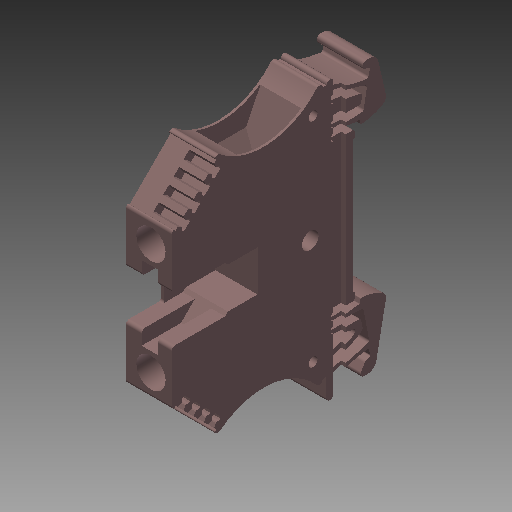
# Autodesk Inventor part: WDU 10 1020300000
Saved by Autodesk Inventor 2019.3 (Build 233278000, 278)
## iProperties
Category: PARTsolutions
Company: WEIDMUELLER
Created: 2018-11-07
Part Number: WDU 10 1020300000
Material: Generic
Catalog Web Link: www.cadenas.de
Description: WDU 10-Feed Through Terminal
Vendor: WEIDMUELLER
Document SubType Name: Modeling
Designer: psadmin
Manufacturer: WEIDMUELLER
Mass: 15.1532 g
Surface Area: 85.6547 cm^2
Volume: 15.1532 cm^3
Density: 1 g/cm^3
Appearance: PSOLRGB-175-140-135
PSOL_IDENT_0: {$CADENAS_DATA\23d-libs\weidmueller\reihenklemmen\w_series\durchgangs_rk\wdu10.prj},174 {VTYP=3D},{N
PSOL_IDENT_1: B=WDU 10 1020300000},{LINA=WDU 10 1020300000},{NN=WDU 10},{DATE=31.03.2017 09:23:17},{GEOMDATE=27.10
PSOL_IDENT_2: .2015 08:25:59},{VERSION=},{LINEID=10},{WBVAR=},{WBNUMERIC=}  {NB=WDU 10 1020300000},{LINA=WDU 10 10
PSOL_IDENT_3: 20300000},{KT=DUMMY},{BEST=1020300000},{BZ=WDU 10},{M=Wemid},{F=beige},{FCODE=0.69,0.55,0.53,0.00}
NN: WDU 10
NT: Feed Through Terminal
NB: WDU 10 1020300000
NBSYN: $BZ. $BEST.
LINA: WDU 10 1020300000
BEST: 1020300000
BZ: WDU 10
M: Wemid
F: beige
SUPPLIER: WEIDMUELLER
ARTICLENO: WDU 10 1020300000
BOMINFO: WDU 10 1020300000
CREATOR: CADENAS GmbH
Title: WDU 10 1020300000
Author: Cadenas PARTsolutions
Comments: Feed Through Terminal
Autodesk Inventor part; units mm, degrees
ref_plane "YZ Plane" through (0, 0, 0) normal (1, 0, 0) x (0, 1, 0)
ref_plane "XZ Plane" through (0, 0, 0) normal (0, 1, 0) x (-1, 0, 0)
ref_plane "XY Plane" through (0, 0, 0) normal (0, 0, 1) x (1, 0, 0)
sketch "Sketch_1" plane through (0, 0, 0) normal (1, 0, 0) x (0, 1, 0)
  line L0 (48.05, 46.25) -> (37.75, 46.25)
  arc A0 (37.75, 46.25) -> (37, 45.5) centre (37.75, 45.5) ccw
  line L1 (37, 45.5) -> (37, 39.25)
  arc A1 (36.5, 38.75) -> (37, 39.25) centre (36.5, 39.25) ccw
  line L2 (36.5, 38.75) -> (27.5, 38.75)
  arc A2 (27, 39.25) -> (27.5, 38.75) centre (27.5, 39.25) ccw
  line L3 (27, 39.25) -> (27, 45.5)
  arc A3 (27, 45.5) -> (26.25, 46.25) centre (26.25, 45.5) ccw
  line L4 (26.25, 46.25) -> (15.95, 46.25)
  arc A4 (15.95, 46.25) -> (15.4144, 46.0251) centre (15.95, 45.5) ccw
  arc A5 (15.4144, 46.0251) -> (15.4159, 45.673) centre (15.5927, 45.8497) ccw
  line L5 (15.4159, 45.673) -> (15.6294, 45.4594)
  line L6 (15.6294, 45.4594) -> (6.7906, 36.6206)
  line L7 (6.7906, 36.6206) -> (6.577, 36.8341)
  arc A6 (6.577, 36.8341) -> (6.2256, 36.8362) centre (6.4003, 36.6573) ccw
  arc A7 (6.2256, 36.8362) -> (6.1668, 35.8284) centre (6.75, 36.3) ccw
  arc A8 (4.2611, 14.9688) -> (6.1668, 35.8284) centre (-5.5492, 26.3819) ccw
  arc A9 (4.2611, 14.9688) -> (4.75, 13.65) centre (4.75, 14.4) ccw
  line L8 (4.75, 13.65) -> (4.75, 12.9)
  line L9 (4.75, 12.9) -> (0.75, 12.9)
  arc A10 (0.75, 12.9) -> (0.4862, 11.4479) centre (0.75, 12.15) ccw
  line L10 (0.4862, 11.4479) -> (1.9437, 10.9003)
  line L11 (1.9437, 10.9003) -> (3.401, 10.9003)
  arc A11 (3.8733, 10.5645) -> (3.401, 10.9003) centre (3.401, 10.4003) ccw
  arc A12 (5.4944, 4.2319) -> (3.8733, 10.5645) centre (-33.9366, -2.4884) ccw
  arc A13 (5.333, 3.774) -> (5.4944, 4.2319) centre (5.0014, 4.1482) ccw
  arc A14 (5.2197, 3.7112) -> (5.333, 3.774) centre (5.1344, 3.9988) ccw
  line L12 (5.2197, 3.7112) -> (4.167, 3.399)
  arc A15 (3.9289, 3.5062) -> (4.167, 3.399) centre (4.1102, 3.5908) ccw
  line L13 (3.9289, 3.5062) -> (3.559, 4.299)
  arc A16 (3.559, 4.299) -> (3.255, 4.632) centre (2.8787, 3.9832) ccw
  line L14 (3.255, 4.632) -> (1.925, 5.4)
  arc A17 (1.925, 5.4) -> (0.8, 4.7505) centre (1.55, 4.7505) ccw
  line L15 (0.8, 4.7505) -> (0.8, 4.05)
  arc A18 (0.8, 4.05) -> (2.4156, 2.0873) centre (2.8, 4.05) ccw
  line L16 (2.4156, 2.0873) -> (12.9502, 0.0242)
  arc A19 (12.9502, 0.0242) -> (14.303, 0.6119) centre (13.2, 1.3) ccw
  arc A20 (14.303, 0.6119) -> (15.7996, 5.2872) centre (5.8187, 5.905) ccw
  arc A21 (15.7996, 5.2872) -> (15.6552, 5.4922) centre (15.6, 5.2999) ccw
  line L17 (15.6552, 5.4922) -> (14.9048, 5.7077)
  arc A22 (14.76, 5.9) -> (14.9048, 5.7077) centre (14.96, 5.9) ccw
  line L18 (14.76, 5.9) -> (14.76, 6.75)
  arc A23 (14.5026, 11.4514) -> (14.76, 6.75) centre (29.4233, 9.9104) ccw
  arc A24 (15, 11.9) -> (14.5026, 11.4514) centre (15, 11.4) ccw
  line L19 (15, 11.9) -> (15.5, 11.9)
  arc A25 (16, 11.4) -> (15.5, 11.9) centre (15.5, 11.4) ccw
  line L20 (16, 11.4) -> (16, 7.25)
  arc A26 (16, 7.25) -> (16.5, 6.75) centre (16.5, 7.25) ccw
  line L21 (16.5, 6.75) -> (17.5, 6.75)
  line L22 (17.5, 6.75) -> (17.8, 7.05)
  line L23 (17.8, 7.05) -> (46.2, 7.05)
  line L24 (46.2, 7.05) -> (46.5, 6.75)
  line L25 (46.5, 6.75) -> (47.5, 6.75)
  arc A27 (47.5, 6.75) -> (48, 7.25) centre (47.5, 7.25) ccw
  line L26 (48, 7.25) -> (48, 11.4)
  arc A28 (48.5, 11.9) -> (48, 11.4) centre (48.5, 11.4) ccw
  line L27 (48.5, 11.9) -> (49, 11.9)
  arc A29 (49.4974, 11.4509) -> (49, 11.9) centre (49, 11.4) ccw
  arc A30 (49.24, 6.7494) -> (49.4974, 11.4509) centre (34.5768, 9.91) ccw
  line L28 (49.24, 6.7494) -> (49.24, 5.9)
  arc A31 (49.0952, 5.7078) -> (49.24, 5.9) centre (49.04, 5.9) ccw
  line L29 (49.0952, 5.7078) -> (48.3444, 5.4921)
  arc A32 (48.3444, 5.4921) -> (48.2004, 5.2878) centre (48.3995, 5.3003) ccw
  arc A33 (48.2004, 5.2878) -> (49.697, 0.6119) centre (58.1813, 5.905) ccw
  arc A34 (49.697, 0.6119) -> (51.0937, 0.0336) centre (50.8, 1.3) ccw
  line L30 (51.0937, 0.0336) -> (58.147, 1.6508)
  arc A35 (58.147, 1.6508) -> (59.7, 3.6004) centre (57.7, 3.6002) ccw
  line L31 (59.7, 3.6004) -> (59.7, 4.25)
  arc A36 (59.7, 4.25) -> (58.95, 5) centre (58.95, 4.25) ccw
  line L32 (58.95, 5) -> (58.6838, 5)
  arc A37 (58.6838, 5) -> (58.2009, 4.6297) centre (58.6838, 4.5) ccw
  line L33 (58.2009, 4.6297) -> (57.9338, 3.6353)
  arc A38 (57.697, 3.492) -> (57.9338, 3.6353) centre (57.7407, 3.6872) ccw
  line L34 (57.697, 3.492) -> (56.4904, 3.762)
  arc A39 (56.1072, 4.3347) -> (56.4904, 3.762) centre (56.6, 4.2499) ccw
  arc A40 (57.8794, 11.0689) -> (56.1072, 4.3347) centre (95.5295, -2.4393) ccw
  arc A41 (58.35, 11.4) -> (57.8794, 11.0689) centre (58.35, 10.9) ccw
  line L35 (58.35, 11.4) -> (59.25, 11.4)
  arc A42 (59.25, 11.4) -> (59.25, 12.9) centre (59.25, 12.15) ccw
  line L36 (59.25, 12.9) -> (59.25, 13.65)
  arc A43 (59.25, 13.65) -> (59.7395, 14.9682) centre (59.25, 14.4) ccw
  arc A44 (57.8338, 35.8292) -> (59.7395, 14.9682) centre (69.5492, 26.3819) ccw
  arc A45 (57.8338, 35.8292) -> (57.7746, 36.836) centre (57.25, 36.3) ccw
  arc A46 (57.7746, 36.836) -> (57.423, 36.8341) centre (57.5997, 36.6573) ccw
  line L37 (57.423, 36.8341) -> (57.2094, 36.6206)
  line L38 (57.2094, 36.6206) -> (48.3706, 45.4594)
  line L39 (48.3706, 45.4594) -> (48.5841, 45.673)
  arc A47 (48.5841, 45.673) -> (48.5856, 46.0251) centre (48.4073, 45.8497) ccw
  arc A48 (48.5856, 46.0251) -> (48.05, 46.25) centre (48.05, 45.5) ccw
  arc A49 (8.5, 11.4) -> (8.0182, 10.7663) centre (8.5, 10.9) ccw
  arc A50 (8.0182, 10.7663) -> (9.6067, 7.0644) centre (22.4721, 14.7768) ccw
  arc A51 (9.6067, 7.0644) -> (10.8714, 7.0301) centre (10.25, 7.45) ccw
  arc A52 (11, 7.9696) -> (10.8714, 7.0301) centre (11.3, 7.45) ccw
  line L40 (11, 7.9696) -> (11, 10.9)
  arc A53 (11, 10.9) -> (10.5, 11.4) centre (10.5, 10.9) ccw
  line L41 (10.5, 11.4) -> (8.5, 11.4)
  arc A54 (55.55, 11.9) -> (55.0535, 11.4588) centre (55.55, 11.4) ccw
  arc A55 (53.9858, 5.5317) -> (55.0535, 11.4588) centre (5.4009, 17.3431) ccw
  arc A56 (53.4019, 5.1597) -> (53.9858, 5.5317) centre (53.5, 5.65) ccw
  line L42 (53.4019, 5.1597) -> (52.4019, 5.3597)
  arc A57 (52, 5.85) -> (52.4019, 5.3597) centre (52.5, 5.85) ccw
  line L43 (52, 5.85) -> (52, 11.4)
  arc A58 (52, 11.4) -> (51.5, 11.9) centre (51.5, 11.4) ccw
  line L44 (51.5, 11.9) -> (51.0523, 11.9)
  arc A59 (51.0523, 11.9) -> (50.5585, 11.4781) centre (51.0523, 11.4) ccw
  arc A60 (50.5585, 11.4781) -> (50.4084, 5.257) centre (73.7984, 7.8051) ccw
  arc A61 (50.4084, 5.257) -> (50.8126, 4.8199) centre (50.9055, 5.3112) ccw
  line L45 (50.8126, 4.8199) -> (54.4786, 4.1269)
  arc A62 (54.4786, 4.1269) -> (55.0409, 4.4461) centre (54.5714, 4.6182) ccw
  arc A63 (55.0409, 4.4461) -> (56.8124, 11.3239) centre (21.3911, 16.7805) ccw
  arc A64 (56.8124, 11.3239) -> (56.3182, 11.9) centre (56.3182, 11.4) ccw
  line L46 (56.3182, 11.9) -> (55.55, 11.9)
  arc A65 (12.5, 11.9) -> (12, 11.4) centre (12.5, 11.4) ccw
  line L47 (12, 11.4) -> (12, 5.85)
  arc A66 (11.5921, 5.3586) -> (12, 5.85) centre (11.5, 5.85) ccw
  line L48 (11.5921, 5.3586) -> (9.9921, 5.0586)
  arc A67 (9.4818, 5.2759) -> (9.9921, 5.0586) centre (9.9, 5.55) ccw
  arc A68 (7.0291, 10.543) -> (9.4818, 5.2759) centre (26.1938, 16.2627) ccw
  arc A69 (7.0291, 10.543) -> (6.55, 10.9) centre (6.55, 10.4) ccw
  line L49 (6.55, 10.9) -> (5.3694, 10.9)
  arc A70 (5.3694, 10.9) -> (4.8818, 10.2893) centre (5.3694, 10.4) ccw
  arc A71 (4.8818, 10.2893) -> (6.5858, 4.0374) centre (78.6169, 27.0276) ccw
  arc A72 (6.5858, 4.0374) -> (7.1536, 3.6979) centre (7.0621, 4.1895) ccw
  line L50 (7.1536, 3.6979) -> (13.1856, 4.8201)
  arc A73 (13.1856, 4.8201) -> (13.5912, 5.2575) centre (13.0941, 5.3117) ccw
  arc A74 (13.5912, 5.2575) -> (13.4421, 11.478) centre (-9.7985, 7.8091) ccw
  arc A75 (13.4421, 11.478) -> (12.9482, 11.9) centre (12.9482, 11.4) ccw
  line L51 (12.9482, 11.9) -> (12.5, 11.9)
  constraints: 152 point on circle, 104 end point, 76 centre point
extrude "Extrusion1" add sketch "Sketch_1" along normal blind 9.9
sketch "Skizze_2" plane through (5.4, 0, 0) normal (1, 0, 0) x (0, 0, -1)
  line L0 (-46.75, 20) -> (-38.75, 20)
  line L1 (-38.75, 20) -> (-38.75, 16.84)
  line L2 (-38.75, 16.84) -> (-46.75, 16.84)
  line L3 (-46.75, 16.84) -> (-46.75, 20)
  line L4 (-46.75, 20) -> (-38.75, 20)
  constraints: 10 end point
revolve "Revolution1" cut sketch "Skizze_2" angle 360 about axis through (5.4, 20, 46.75) along (0, 0, 1)
sketch "Skizze_3" plane through (5.4, 0, 0) normal (1, 0, 0) x (0, 0, -1)
  line L0 (-46.75, 44) -> (-38.75, 44)
  line L1 (-38.75, 44) -> (-38.75, 40.84)
  line L2 (-38.75, 40.84) -> (-46.75, 40.84)
  line L3 (-46.75, 40.84) -> (-46.75, 44)
  line L4 (-46.75, 44) -> (-38.75, 44)
  constraints: 10 end point
revolve "Revolution2" cut sketch "Skizze_3" angle 360 about axis through (5.4, 44, 46.75) along (0, 0, 1)
sketch "Skizze_4" plane through (0.5, 0, 0) normal (1, 0, 0) x (0, 0, -1)
  line L0 (-31.85, 55.5) -> (-26.28, 47.5)
  line L1 (-26.28, 47.5) -> (-22.38, 47.5)
  line L2 (-22.38, 47.5) -> (-17.65, 57.2)
  line L3 (-17.65, 57.2) -> (-31.85, 55.5)
  constraints: 8 end point
extrude "Extrusion2" cut sketch "Skizze_4" along normal blind 8.9
sketch "Skizze_5" plane through (0.5, 0, 0) normal (1, 0, 0) x (0, 0, -1)
  line L0 (-31.85, 8.5) -> (-17.65, 6.8)
  line L1 (-17.65, 6.8) -> (-22.38, 16.5)
  line L2 (-22.38, 16.5) -> (-26.28, 16.5)
  line L3 (-26.28, 16.5) -> (-31.85, 8.5)
  constraints: 8 end point
extrude "Extrusion3" cut sketch "Skizze_5" along normal blind 8.9
sketch "Sketch_5" plane through (0, 0, 23.45) normal (0, 0, 1) x (1, 0, 0)
  line L0 (0.3069, 14.1657) -> (0.5, 13.285)
  line L1 (0.5, 13.285) -> (6.4333, 19.2183)
  line L2 (6.4333, 19.2183) -> (9.4, 13.285)
  line L3 (9.4, 13.285) -> (9.6402, 14.1657)
  line L4 (9.6402, 14.1657) -> (9.6402, 49.3357)
  line L5 (9.6402, 49.3357) -> (9.4, 50.715)
  line L6 (9.4, 50.715) -> (6.4333, 44.7817)
  line L7 (6.4333, 44.7817) -> (0.5, 50.715)
  line L8 (0.5, 50.715) -> (0.3069, 50.0567)
  line L9 (0.3069, 50.0567) -> (0.3069, 14.1657)
  constraints: 20 end point
extrude "Extrusion4" add sketch "Sketch_5" along normal mid plane 10
sketch "Sketch_4" plane through (5.15, 0, 0) normal (1, 0, 0) x (0, 0, -1)
  line L0 (-47.25, 40) -> (-47.25, 24)
  line L1 (-47.25, 24) -> (-37.75, 24)
  line L2 (-37.75, 24) -> (-34.15, 27.6)
  line L3 (-34.15, 27.6) -> (-27.75, 27.6)
  line L4 (-27.75, 27.6) -> (-27.75, 36.4)
  line L5 (-27.75, 36.4) -> (-34.15, 36.4)
  line L6 (-34.15, 36.4) -> (-37.75, 40)
  line L7 (-37.75, 40) -> (-47.25, 40)
  constraints: 16 end point
extrude "Extrusion5" cut sketch "Sketch_4" along normal mid plane 3.55
sketch "Sketch_2" plane through (9.9, 0, 0) normal (1, 0, 0) x (0, 0, -1)
  line L0 (-47.25, 37) -> (-47.25, 27)
  line L1 (-47.25, 27) -> (-34.75, 27)
  line L2 (-34.75, 27) -> (-34.15, 27.6)
  line L3 (-34.15, 27.6) -> (-27.75, 27.6)
  line L4 (-27.75, 27.6) -> (-27.75, 36.4)
  line L5 (-27.75, 36.4) -> (-34.15, 36.4)
  line L6 (-34.15, 36.4) -> (-34.75, 37)
  line L7 (-34.75, 37) -> (-47.25, 37)
  constraints: 16 end point
extrude "Extrusion6" cut sketch "Sketch_2" against normal blind 9.1
sketch "Sketch_3" plane through (4.55, 0, 0) normal (1, 0, 0) x (0, 0, -1)
  line L0 (-50.2151, 49.9527) -> (-48.7516, 12.801)
  line L1 (-48.7516, 12.801) -> (-38.528, 4.5188)
  line L2 (-38.528, 4.5188) -> (-36.7355, 8.0369)
  line L3 (-36.7355, 8.0369) -> (-36.5941, 8.1783)
  line L4 (-36.5941, 8.1783) -> (-36.0107, 8.1783)
  line L5 (-36.0107, 8.1783) -> (-35.7721, 8.4169)
  line L6 (-35.7721, 8.4169) -> (-35.7721, 8.8412)
  line L7 (-35.7721, 8.8412) -> (-36.8327, 9.9019)
  line L8 (-36.8327, 9.9019) -> (-37.257, 9.9019)
  line L9 (-37.257, 9.9019) -> (-37.4956, 9.6632)
  line L10 (-37.4956, 9.6632) -> (-37.4956, 9.0798)
  line L11 (-37.4956, 9.0798) -> (-37.637, 8.9384)
  line L12 (-37.637, 8.9384) -> (-39.0655, 8.2106)
  line L13 (-39.0655, 8.2106) -> (-39.6679, 8.7757)
  line L14 (-39.6679, 8.7757) -> (-38.9275, 10.2289)
  line L15 (-38.9275, 10.2289) -> (-38.7861, 10.3703)
  line L16 (-38.7861, 10.3703) -> (-38.2027, 10.3703)
  line L17 (-38.2027, 10.3703) -> (-37.9641, 10.609)
  line L18 (-37.9641, 10.609) -> (-37.9641, 11.0332)
  line L19 (-37.9641, 11.0332) -> (-39.0247, 12.0939)
  line L20 (-39.0247, 12.0939) -> (-39.449, 12.0939)
  line L21 (-39.449, 12.0939) -> (-39.6877, 11.8552)
  line L22 (-39.6877, 11.8552) -> (-39.6877, 11.2719)
  line L23 (-39.6877, 11.2719) -> (-39.8291, 11.1305)
  line L24 (-39.8291, 11.1305) -> (-41.1372, 10.4639)
  line L25 (-41.1372, 10.4639) -> (-41.7545, 11.1748)
  line L26 (-41.7545, 11.1748) -> (-41.1195, 12.4209)
  line L27 (-41.1195, 12.4209) -> (-40.9781, 12.5623)
  line L28 (-40.9781, 12.5623) -> (-40.3948, 12.5623)
  line L29 (-40.3948, 12.5623) -> (-40.1561, 12.801)
  line L30 (-40.1561, 12.801) -> (-40.1561, 13.2253)
  line L31 (-40.1561, 13.2253) -> (-41.2168, 14.2859)
  line L32 (-41.2168, 14.2859) -> (-41.641, 14.2859)
  line L33 (-41.641, 14.2859) -> (-41.8797, 14.0473)
  line L34 (-41.8797, 14.0473) -> (-41.8797, 13.4639)
  line L35 (-41.8797, 13.4639) -> (-42.0211, 13.3225)
  line L36 (-42.0211, 13.3225) -> (-43.3692, 12.6356)
  line L37 (-43.3692, 12.6356) -> (-43.9752, 13.3106)
  line L38 (-43.9752, 13.3106) -> (-43.3116, 14.613)
  line L39 (-43.3116, 14.613) -> (-43.1702, 14.7544)
  line L40 (-43.1702, 14.7544) -> (-42.5868, 14.7544)
  line L41 (-42.5868, 14.7544) -> (-42.3481, 14.993)
  line L42 (-42.3481, 14.993) -> (-42.3481, 15.4173)
  line L43 (-42.3481, 15.4173) -> (-43.4088, 16.4779)
  line L44 (-43.4088, 16.4779) -> (-43.8331, 16.4779)
  line L45 (-43.8331, 16.4779) -> (-44.0717, 16.2393)
  line L46 (-44.0717, 16.2393) -> (-44.0717, 15.6559)
  line L47 (-44.0717, 15.6559) -> (-44.2131, 15.5145)
  line L48 (-44.2131, 15.5145) -> (-46.5212, 14.3385)
  line L49 (-46.5212, 14.3385) -> (-46.7415, 49.7737)
  line L50 (-46.7415, 49.7737) -> (-44.2131, 48.4855)
  line L51 (-44.2131, 48.4855) -> (-44.0717, 48.3441)
  line L52 (-44.0717, 48.3441) -> (-44.0717, 47.7607)
  line L53 (-44.0717, 47.7607) -> (-43.8331, 47.5221)
  line L54 (-43.8331, 47.5221) -> (-43.4088, 47.5221)
  line L55 (-43.4088, 47.5221) -> (-42.3481, 48.5827)
  line L56 (-42.3481, 48.5827) -> (-42.3481, 49.007)
  line L57 (-42.3481, 49.007) -> (-42.5868, 49.2456)
  line L58 (-42.5868, 49.2456) -> (-43.1702, 49.2456)
  line L59 (-43.1702, 49.2456) -> (-43.3116, 49.387)
  line L60 (-43.3116, 49.387) -> (-44.0128, 50.7632)
  line L61 (-44.0128, 50.7632) -> (-43.3726, 51.3661)
  line L62 (-43.3726, 51.3661) -> (-42.0211, 50.6775)
  line L63 (-42.0211, 50.6775) -> (-41.8797, 50.5361)
  line L64 (-41.8797, 50.5361) -> (-41.8797, 49.9527)
  line L65 (-41.8797, 49.9527) -> (-41.641, 49.7141)
  line L66 (-41.641, 49.7141) -> (-41.2168, 49.7141)
  line L67 (-41.2168, 49.7141) -> (-40.1561, 50.7747)
  line L68 (-40.1561, 50.7747) -> (-40.1561, 51.199)
  line L69 (-40.1561, 51.199) -> (-40.3948, 51.4377)
  line L70 (-40.3948, 51.4377) -> (-40.9781, 51.4377)
  line L71 (-40.9781, 51.4377) -> (-41.1195, 51.5791)
  line L72 (-41.1195, 51.5791) -> (-41.926, 53.1619)
  line L73 (-41.926, 53.1619) -> (-41.3958, 53.6678)
  line L74 (-41.3958, 53.6678) -> (-39.8291, 52.8696)
  line L75 (-39.8291, 52.8696) -> (-39.6877, 52.7281)
  line L76 (-39.6877, 52.7281) -> (-39.6877, 52.1448)
  line L77 (-39.6877, 52.1448) -> (-39.449, 51.9061)
  line L78 (-39.449, 51.9061) -> (-39.0247, 51.9061)
  line L79 (-39.0247, 51.9061) -> (-37.9641, 52.9668)
  line L80 (-37.9641, 52.9668) -> (-37.9641, 53.391)
  line L81 (-37.9641, 53.391) -> (-38.2027, 53.6297)
  line L82 (-38.2027, 53.6297) -> (-38.7861, 53.6297)
  line L83 (-38.7861, 53.6297) -> (-38.9275, 53.7711)
  line L84 (-38.9275, 53.7711) -> (-39.7094, 55.3057)
  line L85 (-39.7094, 55.3057) -> (-39.1789, 55.8472)
  line L86 (-39.1789, 55.8472) -> (-37.637, 55.0616)
  line L87 (-37.637, 55.0616) -> (-37.4956, 54.9202)
  line L88 (-37.4956, 54.9202) -> (-37.4956, 54.3368)
  line L89 (-37.4956, 54.3368) -> (-37.257, 54.0982)
  line L90 (-37.257, 54.0982) -> (-36.8327, 54.0982)
  line L91 (-36.8327, 54.0982) -> (-35.7721, 55.1588)
  line L92 (-35.7721, 55.1588) -> (-35.7721, 55.5831)
  line L93 (-35.7721, 55.5831) -> (-36.0107, 55.8217)
  line L94 (-36.0107, 55.8217) -> (-36.5941, 55.8217)
  line L95 (-36.5941, 55.8217) -> (-36.7355, 55.9631)
  line L96 (-36.7355, 55.9631) -> (-38.9183, 60.2472)
  line L97 (-38.9183, 60.2472) -> (-50.2151, 49.9527)
  constraints: 196 end point
extrude "Extrusion7" cut sketch "Sketch_3" along normal blind 6.35
sketch "Sketch_6" plane through (0, 0, 0) normal (0, 1, 0) x (-1, 0, 0)
  line L0 (-8.9, 11.35) -> (-9.9, 11.35)
  line L1 (-9.9, 11.35) -> (-9.9, 8.7)
  line L2 (-9.9, 8.7) -> (-8.9, 8.7)
  line L3 (-8.9, 8.7) -> (-8.9, 11.35)
  constraints: 8 end point
extrude "Extrusion8" cut sketch "Sketch_6" along normal blind 70
sketch "Sketch11" plane through (0, 0, 0) normal (-1, 0, 0) x (0, 0, 1)
  point P0 (15.75, 9)
hole "Hole1" at (0, 9, 15.75) direction (1, 0, 0) diameter 2.56 depth 2.65
sketch "Sketch12" plane through (0, 0, 0) normal (-1, 0, 0) x (0, 0, 1)
  point P0 (15.75, 55)
hole "Hole2" at (0, 55, 15.75) direction (1, 0, 0) diameter 2.56 depth 2.65
sketch "Sketch13" plane through (0, 0, 0) normal (-1, 0, 0) x (0, 0, 1)
  point P0 (16.35, 32)
hole "Hole3" at (0, 32, 16.35) direction (1, 0, 0) diameter 3.6 depth 10
sketch "Sketch14" plane through (9.9, 0, 0) normal (1, 0, 0) x (0, 0, -1)
  point P0 (-15.75, 9)
hole "Hole4" at (9.9, 9, 15.75) direction (-1, 0, 0) diameter 1.98 depth 2.625
sketch "Sketch15" plane through (9.9, 0, 0) normal (1, 0, 0) x (0, 0, -1)
  point P0 (-15.75, 55)
hole "Hole5" at (9.9, 55, 15.75) direction (-1, 0, 0) diameter 1.98 depth 2.625
body "Solid1"
